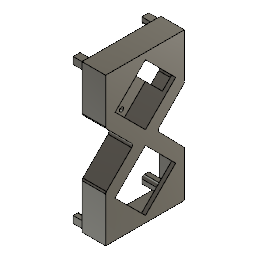
Hourglass v10 (Autodesk Fusion 360 design; units mm, degrees)
Autodesk Fusion 360 part; units mm, degrees
sketch "Sketch4" plane through (0, 0, 0) normal (1, 0, 0) x (0, 1, 0)
  line L0 (-60, 0) -> (-60, 35)
  line L1 (-60, 35) -> (0, 35)
  line L2 (0, 35) -> (0, 0)
  line L3 (-60, 0) -> (-38.7868, -21.2132)
  line L4 (-29.7466, 65.753) -> (-29.7466, -62.8744) construction
  line L5 (0, 0) -> (-20.7064, -21.2132)
  line L6 (-20.7064, -21.2132) -> (-38.7868, -21.2132)
  line L7 (-29.7466, 30) -> (-6.7656, 7.019)
  line L8 (-6.7656, 7.019) -> (-29.7466, -15.9619)
  line L9 (-29.7466, -15.9619) -> (-52.7276, 7.019)
  line L10 (-52.7276, 7.019) -> (-29.7466, 30)
  line L11 (-60, -42.4264) -> (-60, -77.4264)
  line L12 (-52.7276, -49.4454) -> (-29.7466, -72.4264)
  line L13 (-29.7466, -72.4264) -> (-6.7656, -49.4454)
  line L14 (0, -77.4264) -> (0, -42.4264)
  line L15 (-60, -42.4264) -> (-38.7868, -21.2132)
  line L16 (-6.7656, -49.4454) -> (-29.7466, -26.4645)
  line L17 (-29.7466, -26.4645) -> (-52.7276, -49.4454)
  line L18 (0, -42.4264) -> (-20.7064, -21.2132)
  line L19 (-60, -77.4264) -> (0, -77.4264)
  line L20 (-29.7466, -108.1794) -> (-29.7466, 20.448) construction
  line L21 (0, 0) -> (-13.7847, 0)
  line L22 (-45.7085, 0) -> (-60, 0)
  line L23 (0, -42.4264) -> (-13.7847, -42.4264)
  line L24 (-45.7085, -42.4264) -> (-60, -42.4264)
  line L25 (-58.8, 0.4971) -> (-58.8, 33.8)
  line L26 (-58.8, 33.8) -> (-1.2, 33.8)
  line L27 (-1.2, 33.8) -> (-1.2, 0.4886)
  line L28 (-1.2, 0.4886) -> (-22.3833, -21.2132)
  line L29 (-1.2, -42.915) -> (-22.3833, -21.2132)
  line L30 (-1.2, -76.2264) -> (-1.2, -42.915)
  line L31 (-58.8, -76.2264) -> (-1.2, -76.2264)
  line L32 (-58.8, -42.9235) -> (-58.8, -76.2264)
  line L33 (-58.8, -42.9235) -> (-37.0897, -21.2132)
  line L34 (-58.8, 0.4971) -> (-37.0897, -21.2132)
  line L35 (-29.7466, -17.659) -> (-54.4246, 7.019)
  line L36 (-54.4246, 7.019) -> (-29.7466, 31.6971)
  line L37 (-29.7466, 31.6971) -> (-5.0686, 7.019)
  line L38 (-5.0686, 7.019) -> (-29.7466, -17.659)
  line L39 (-29.7466, -24.7674) -> (-54.4246, -49.4454)
  line L40 (-54.4246, -49.4454) -> (-29.7466, -74.1235)
  line L41 (-29.7466, -74.1235) -> (-5.0686, -49.4454)
  line L42 (-5.0686, -49.4454) -> (-29.7466, -24.7674)
  line L43 (-29.7466, 30) -> (-30.5951, 30.8485)
  line L44 (-6.7656, 7.019) -> (-5.9171, 6.1705)
  line L45 (-36.8177, 22.9289) -> (-37.6662, 23.7775)
  line L46 (-13.8367, -0.052) -> (-12.9882, -0.9006)
  circle A0 centre (-31.9386, -9.5273) radius 1.6
  circle A1 centre (-46.2929, 4.827) radius 1.6
  line L47 (-6.7656, -49.4454) -> (-5.9171, -48.5969)
  line L48 (-29.7466, -72.4264) -> (-30.5951, -73.2749)
  line L49 (-13.8367, -42.3744) -> (-12.9882, -41.5258)
  line L50 (-36.8177, -65.3553) -> (-37.6662, -66.2039)
  circle A2 centre (-31.9386, -32.8991) radius 1.6
  circle A3 centre (-46.2929, -47.2534) radius 1.6
  point P0 (0, -42.4264)
  dimension "d13" = 60
  dimension "d14" = 35
  dimension "d15" = 30
  dimension "d16" = 45
  dimension "d17" = 32.5
  dimension "d18" = 45
  dimension "d19" = 5
  dimension "d20" = 32.5
  dimension "d33" = 1.2
  dimension "d34" = -1.2
  dimension "d35" = 1.2
  dimension "d50" = 10
  dimension "d51" = 10
  dimension "d58" = 3.2
  dimension "d59" = 3
  dimension "d60" = 6.1
  dimension "d61" = 3.2
  dimension "d62" = 6.1
  dimension "d63" = 3
  dimension "d66" = 10
  dimension "d67" = 10
  dimension "d72" = 3.2
  dimension "d73" = 3.2
  dimension "d74" = 6.1
  dimension "d75" = 3
  dimension "d76" = 3
  dimension "d77" = 6.1
  constraint horizontal L21
  constraint vertical L0
  constraint horizontal L1
  constraint vertical L2
  constraint coincident L2.end L5.start
  constraint perpendicular L1 L4
  constraint symmetric L3.end L4 L5.end
  constraint perpendicular L7 L8
  constraint parallel L7 L9
  constraint parallel L8 L10
  constraint coincident L4 L7.start
  constraint symmetric L2.end L6 L14.end
  constraint symmetric L2.end L6 P0
  constraint symmetric L0.start L6 L11.start
  constraint symmetric L0.end L6 L11.end
  constraint symmetric L1.end L6 L14.start
  constraint symmetric L3.end L6 L15.end
  constraint symmetric L4.start L6 L20.start
  constraint symmetric L4.end L6 L20.end
  constraint symmetric L5.end L6 L18.end
  constraint symmetric L6 L7.start L12.end
  constraint symmetric L6 L7.end L13.end
  constraint symmetric L6 L8.end L16.end
  constraint symmetric L6 L9.end L12.start
  constraint coincident L8 L21.end
  constraint collinear L21 L22
  constraint coincident L9 L22.start
  constraint coincident L16 L23.end
  constraint collinear L23 L24
  constraint coincident L17 L24.start
  constraint coincident L36 L43.end
  constraint perpendicular L36 L43
  constraint coincident L38 L44.end
  constraint perpendicular L38 L44
  constraint coincident L10 L45.start
  constraint coincident L36 L45.end
  constraint perpendicular L36 L45
  constraint coincident L8 L46.start
  constraint coincident L38 L46.end
  constraint perpendicular L38 L46
  constraint coincident L42 L47.end
  constraint perpendicular L42 L47
  constraint coincident L40 L48.end
  constraint perpendicular L40 L48
  constraint coincident L16 L49.start
  constraint coincident L42 L49.end
  constraint perpendicular L42 L49
  constraint coincident L12 L50.start
  constraint coincident L40 L50.end
  constraint perpendicular L40 L50
  measures "d13" distance of L2.end L0.start
  measures "d14" distance of L2.end L1.end
  measures "d15" distance of L0.start L3.end
  measures "d16" angle of L3 L21
  measures "d17" distance of L7.start L9.end
  measures "d18" angle of L4 L7
  measures "d19" distance of L1 L7.start
  measures "d20" distance of L7.start L7.end
  measures "d50" distance of L43 L45
  measures "d51" distance of L44 L46
  measures "d58" diameter of A0
  measures "d59" distance of L9 A0.centre
  measures "d60" distance of L8 A0.centre
  measures "d61" diameter of A1
  measures "d62" distance of L10 A1.centre
  measures "d63" distance of L9 A1.centre
  measures "d66" distance of L47 L49
  measures "d67" distance of L48 L50
  measures "d72" diameter of A2
  measures "d73" diameter of A3
  measures "d74" distance of L16 A2.centre
  measures "d75" distance of L17 A2.centre
  measures "d76" distance of L17 A3.centre
  measures "d77" distance of L12 A3.centre
extrude "Extrude2" add sketch "Sketch4" along normal blind 18 contours L3 L6 L22 L34 | L0 L1 L2 L21 L22 L25 L26 L27 L28 L34 | L6 L15 L24 L33 | L21 L22 L25 L26 L27 L28 L34 L35 L36 L37 L38 | L6 L21 L22 L28 L34 L35 L38 | L6 L23 L24 L29 L33 L39 L42 | L11 L14 L19 L23 L24 L29 L30 L31 L32 L33 | L9 L10 L22 L35 L36 L45 | L8 L9 L22 L35 L38 L46 | L5 L6 L21 L28 | L6 L18 L23 L29 | L23 L24 L29 L30 L31 L32 L33 L39 L40 L41 L42 | L16 L17 L24 L39 L42 L49 | L12 L17 L24 L39 L40 L50 | L8 L21 L38 L46 | L10 L36 L43 L45 | L8 L21 L38 L44 | L16 L23 L42 L47 | L16 L23 L42 L49 | L7 L36 L37 L38 L43 L44 | L13 L40 L41 L42 L47 L48 | L12 L40 L48 L50 makes body 1
extrude "Extrude3" add sketch "Sketch4" along normal blind 2 contours L12 L13 L16 L17 | A2 | A3 bodies 1
extrude "Extrude4" add sketch "Sketch4" along normal blind 2 contours L7 L8 L9 L10 | A0 | A1 bodies 1
fillet "Fillet1" radius 2 6 edges at (9, -38.7868, -21.2132) (9, -60, -42.4264) (9, -60, 0) (9, -20.7064, -21.2132) (9, 0, 0) (9, 0, -42.4264) on bodies 1
sketch "Sketch5" plane through (2, 0, 0) normal (1, 0, 0) x (0, 1, 0)
  line L0 (-52.7276, 7.019) -> (-29.7466, -15.9619)
  line L1 (-29.7466, -15.9619) -> (-6.7656, 7.019)
  line L2 (-6.7656, 7.019) -> (-29.7466, 30)
  line L3 (-29.7466, 30) -> (-52.7276, 7.019)
  line L4 (-36.8177, 22.9289) -> (-13.8367, -0.052)
  dimension "d29" = 10
  constraint coincident L3 L4.start
  constraint coincident L1 L4.end
  constraint perpendicular L1 L4
  measures "d29" distance of L2 L4
sketch "Sketch7" plane through (2, 0, 0) normal (1, 0, 0) x (0, 1, 0)
  line L0 (-29.7466, -26.4645) -> (-52.7276, -49.4454)
  line L1 (-52.7276, -49.4454) -> (-29.7466, -72.4264)
  line L2 (-29.7466, -72.4264) -> (-6.7656, -49.4454)
  line L3 (-6.7656, -49.4454) -> (-29.7466, -26.4645)
  line L4 (-13.8367, -42.3744) -> (-36.8177, -65.3553)
  dimension "d30" = 10
  constraint coincident L3 L4.start
  constraint perpendicular L1 L4
  constraint coincident L1 L4.end
  measures "d30" distance of L2 L4
extrude "Extrude5" cut sketch "Sketch7" sketch "Sketch5" against normal blind 2 contours L1 L2 L3 L4 of sketch 2 contours L1 L2 L3 L4 bodies 1
extrude "Extrude6" cut sketch "Sketch4" along normal blind 15 contours L21 L22 L25 L26 L27 L28 L34 L35 L36 L37 L38 | L6 L21 L22 L28 L34 L35 L38 | L6 L23 L24 L29 L33 L39 L42 | L23 L24 L29 L30 L31 L32 L33 L39 L40 L41 L42 bodies 1
extrude "Extrude8" cut sketch "Sketch4" along normal blind 15 contours L7 L36 L37 L38 L43 L44 bodies 1
fillet "Fillet4" radius 2 4 edges at (7.5, -30.5951, 30.8485) (7.5, -5.9171, 6.1705) (7.5, -54.4246, 7.019) (7.5, -29.7466, -17.659) on bodies 1
fillet "Fillet5" radius 2 2 edges at (7.5, -22.3833, -21.2132) (7.5, -37.0897, -21.2132) on bodies 1
extrude "Extrude9" cut sketch "Sketch4" along normal blind 15 contours L10 L36 L43 L45 bodies 1
extrude "Extrude10" cut sketch "Sketch4" along normal blind 15 contours L8 L21 L38 L44 bodies 1
extrude "Extrude11" cut sketch "Sketch4" along normal blind 15 contours L8 L21 L38 L46 | L8 L21 L38 L44 bodies 1
extrude "Extrude12" cut sketch "Sketch4" along normal blind 2 contours A0 | A1 bodies 1
extrude "Extrude13" cut sketch "Sketch4" along normal blind 15 contours L16 L23 L42 L47 | L16 L23 L42 L49 | L13 L40 L41 L42 L47 L48 | L12 L40 L48 L50 bodies 1
fillet "Fillet6" radius 2 2 edges at (7.5, -29.7466, -24.7674) (7.5, -54.4246, -49.4454) on bodies 1
extrude "Extrude14" cut sketch "Sketch4" along normal blind 2 contours A2 | A3 bodies 1
sketch "Sketch8" plane through (15, 0, 0) normal (-1, 0, 0) x (0, -1, 0)
  line L0 (58.8, 0.4971) -> (58.8, 33.8)
  line L1 (58.8, 33.8) -> (1.2, 33.8)
  line L2 (1.2, 33.8) -> (1.2, 0.4886)
  line L3 (1.2, 0.4886) -> (21.0197, -19.8162)
  arc A0 (21.0197, -22.6102) -> (21.0197, -19.8162) centre (19.5885, -21.2132) ccw
  line L4 (21.0197, -22.6102) -> (1.2, -42.915)
  line L5 (1.2, -42.915) -> (1.2, -76.2264)
  line L6 (1.2, -76.2264) -> (58.8, -76.2264)
  line L7 (58.8, -76.2264) -> (58.8, -42.9235)
  line L8 (58.8, -42.9235) -> (38.504, -22.6274)
  arc A1 (38.504, -19.799) -> (38.504, -22.6274) centre (39.9182, -21.2132) ccw
  line L9 (38.504, -19.799) -> (58.8, 0.4971)
  line L10 (53.0104, -50.8597) -> (37.6662, -66.2039)
  line L11 (37.6662, -66.2039) -> (36.8177, -65.3553)
  line L12 (36.8177, -65.3553) -> (29.7466, -72.4264)
  line L13 (29.7466, -72.4264) -> (6.7656, -49.4454)
  line L14 (6.7656, -49.4454) -> (13.8367, -42.3744)
  line L15 (13.8367, -42.3744) -> (12.9882, -41.5258)
  line L16 (12.9882, -41.5258) -> (28.3324, -26.1816)
  arc A2 (31.1608, -26.1816) -> (28.3324, -26.1816) centre (29.7466, -27.5958) ccw
  line L17 (31.1608, -26.1816) -> (53.0104, -48.0312)
  arc A3 (53.0104, -50.8597) -> (53.0104, -48.0312) centre (51.5962, -49.4454) ccw
  line L18 (13.8367, -0.052) -> (6.7656, 7.019)
  line L19 (6.7656, 7.019) -> (29.7466, 30)
  line L20 (29.7466, 30) -> (36.8177, 22.9289)
  line L21 (36.8177, 22.9289) -> (37.6662, 23.7775)
  line L22 (37.6662, 23.7775) -> (53.0104, 8.4332)
  arc A4 (53.0104, 5.6048) -> (53.0104, 8.4332) centre (51.5962, 7.019) ccw
  line L23 (53.0104, 5.6048) -> (31.1608, -16.2448)
  arc A5 (28.3324, -16.2448) -> (31.1608, -16.2448) centre (29.7466, -14.8306) ccw
  line L24 (28.3324, -16.2448) -> (12.9882, -0.9006)
  line L25 (12.9882, -0.9006) -> (13.8367, -0.052)
  line L26 (1.2, 33.8) -> (6.6, 33.8)
  line L27 (6.6, 33.8) -> (6.6, 28.4)
  line L28 (6.6, 28.4) -> (1.2, 28.4)
  line L29 (1.2, 28.4) -> (1.2, 33.8)
  line L30 (58.8, 33.8) -> (53.4, 33.8)
  line L31 (53.4, 33.8) -> (53.4, 28.4)
  line L32 (53.4, 28.4) -> (58.8, 28.4)
  line L33 (58.8, 28.4) -> (58.8, 33.8)
  line L34 (58.8, -76.2264) -> (53.4, -76.2264)
  line L35 (53.4, -76.2264) -> (53.4, -70.8264)
  line L36 (53.4, -70.8264) -> (58.8, -70.8264)
  line L37 (58.8, -70.8264) -> (58.8, -76.2264)
  line L38 (1.2, -76.2264) -> (6.6, -76.2264)
  line L39 (6.6, -76.2264) -> (6.6, -70.8264)
  line L40 (6.6, -70.8264) -> (1.2, -70.8264)
  line L41 (1.2, -70.8264) -> (1.2, -76.2264)
  dimension "d80" = 5.4
  dimension "d81" = 5.4
  dimension "d82" = 5.4
  dimension "d83" = 5.4
  dimension "d84" = 5.4
  dimension "d85" = 5.4
  dimension "d86" = 5.4
  dimension "d87" = 5.4
  constraint horizontal L26
  constraint vertical L27
  constraint horizontal L28
  constraint vertical L29
  constraint coincident L1.end L2.start
  constraint horizontal L30
  constraint vertical L31
  constraint horizontal L32
  constraint vertical L33
  constraint coincident L0.end L1.start
  constraint horizontal L34
  constraint vertical L35
  constraint horizontal L36
  constraint vertical L37
  constraint coincident L6.end L7.start
  constraint horizontal L38
  constraint vertical L39
  constraint horizontal L40
  constraint vertical L41
  constraint coincident L5.end L6.start
  measures "d80" distance of L1.end L26.end
  measures "d81" distance of L1.end L28.end
  measures "d82" distance of L0.end L30.end
  measures "d83" distance of L0.end L32.end
  measures "d84" distance of L6.end L34.end
  measures "d85" distance of L6.end L36.end
  measures "d86" distance of L5.end L38.end
  measures "d87" distance of L5.end L40.end
extrude "Extrude15" add sketch "Sketch8" along normal blind 15 contours L0 L1 L30 L31 L32 L33 | L1 L2 L26 L27 L28 L29 | L6 L7 L34 L35 L36 L37 | L5 L6 L38 L39 L40 L41 bodies 1
sketch "Sketch9" plane through (0, 0, 0) normal (-1, 0, 0) x (0, -1, 0)
  arc A0 (38.504, -19.799) -> (38.504, -22.6274) centre (39.9182, -21.2132) ccw
  line L0 (38.504, -22.6274) -> (58.8, -42.9235)
  line L1 (58.8, -42.9235) -> (58.8, -70.8264)
  line L2 (58.8, -70.8264) -> (53.4, -70.8264)
  line L3 (53.4, -70.8264) -> (53.4, -76.2264)
  line L4 (53.4, -76.2264) -> (6.6, -76.2264)
  line L5 (6.6, -76.2264) -> (6.6, -70.8264)
  line L6 (6.6, -70.8264) -> (1.2, -70.8264)
  line L7 (1.2, -70.8264) -> (1.2, -42.915)
  line L8 (1.2, -42.915) -> (21.0197, -22.6102)
  arc A1 (21.0197, -22.6102) -> (21.0197, -19.8162) centre (19.5885, -21.2132) ccw
  line L9 (21.0197, -19.8162) -> (1.2, 0.4886)
  line L10 (1.2, 0.4886) -> (1.2, 28.4)
  line L11 (1.2, 28.4) -> (6.6, 28.4)
  line L12 (6.6, 28.4) -> (6.6, 33.8)
  line L13 (6.6, 33.8) -> (53.4, 33.8)
  line L14 (53.4, 33.8) -> (53.4, 28.4)
  line L15 (53.4, 28.4) -> (58.8, 28.4)
  line L16 (58.8, 28.4) -> (58.8, 0.4971)
  line L17 (58.8, 0.4971) -> (38.504, -19.799)
  arc A2 (0.5688, -41.8437) -> (0, -43.2407) centre (2, -43.2407) ccw
  line L18 (0, -43.2407) -> (0, -77.4264)
  line L19 (0, -77.4264) -> (60, -77.4264)
  line L20 (60, -77.4264) -> (60, -43.2548)
  arc A3 (60, -43.2548) -> (59.4142, -41.8406) centre (58, -43.2548) ccw
  line L21 (59.4142, -41.8406) -> (40.201, -22.6274)
  arc A4 (40.201, -19.799) -> (40.201, -22.6274) centre (41.6152, -21.2132) ccw
  line L22 (40.201, -19.799) -> (59.4142, -0.5858)
  arc A5 (59.4142, -0.5858) -> (60, 0.8284) centre (58, 0.8284) ccw
  line L23 (60, 0.8284) -> (60, 35)
  line L24 (60, 35) -> (0, 35)
  line L25 (0, 35) -> (0, 0.8143)
  arc A6 (0, 0.8143) -> (0.5688, -0.5827) centre (2, 0.8143) ccw
  line L26 (0.5688, -0.5827) -> (19.3428, -19.8162)
  arc A7 (19.3428, -22.6102) -> (19.3428, -19.8162) centre (17.9116, -21.2132) ccw
  line L27 (19.3428, -22.6102) -> (0.5688, -41.8437)
  circle A8 centre (3.9, 31.1) radius 1.5
  circle A9 centre (56.1, 31.1) radius 1.5
  circle A10 centre (56.1, -73.5264) radius 1.5
  circle A11 centre (3.9, -73.5264) radius 1.5
  line L28 (6.6, 28.4) -> (1.2, 28.4)
  line L29 (1.2, 28.4) -> (1.2, 33.8)
  line L30 (1.2, 33.8) -> (6.6, 33.8)
  line L31 (6.6, 33.8) -> (6.6, 28.4)
  line L32 (53.4, 28.4) -> (58.8, 28.4)
  line L33 (58.8, 28.4) -> (58.8, 33.8)
  line L34 (58.8, 33.8) -> (53.4, 33.8)
  line L35 (53.4, 33.8) -> (53.4, 28.4)
  line L36 (53.4, -70.8264) -> (58.8, -70.8264)
  line L37 (58.8, -70.8264) -> (58.8, -76.2264)
  line L38 (58.8, -76.2264) -> (53.4, -76.2264)
  line L39 (53.4, -76.2264) -> (53.4, -70.8264)
  line L40 (6.6, -70.8264) -> (1.2, -70.8264)
  line L41 (1.2, -70.8264) -> (1.2, -76.2264)
  line L42 (1.2, -76.2264) -> (6.6, -76.2264)
  line L43 (6.6, -76.2264) -> (6.6, -70.8264)
  dimension "d90" = 3
  dimension "d91" = 2.7
  dimension "d92" = 2.7
  dimension "d93" = 3
  dimension "d94" = 2.7
  dimension "d95" = 2.7
  dimension "d96" = 3
  dimension "d97" = 2.7
  dimension "d98" = 2.7
  dimension "d99" = 3
  dimension "d100" = 2.7
  dimension "d101" = 2.7
  dimension "d195" = 5.4
  dimension "d196" = 5.4
  dimension "d197" = 5.4
  dimension "d198" = 5.4
  dimension "d199" = 5.4
  dimension "d200" = 5.4
  dimension "d201" = 5.4
  dimension "d202" = 5.4
  constraint horizontal L28
  constraint vertical L29
  constraint horizontal L30
  constraint vertical L31
  constraint coincident L11.end L12.start
  constraint horizontal L32
  constraint vertical L33
  constraint horizontal L34
  constraint vertical L35
  constraint coincident L14.end L15.start
  constraint horizontal L36
  constraint vertical L37
  constraint horizontal L38
  constraint vertical L39
  constraint coincident L2.end L3.start
  constraint horizontal L40
  constraint vertical L41
  constraint horizontal L42
  constraint vertical L43
  constraint coincident L5.end L6.start
  measures "d90" diameter of A8
  measures "d91" distance of L12 A8.centre
  measures "d92" distance of L11 A8.centre
  measures "d93" diameter of A9
  measures "d94" distance of L14 A9.centre
  measures "d95" distance of L15 A9.centre
  measures "d96" diameter of A10
  measures "d97" distance of L3 A10.centre
  measures "d98" distance of L2 A10.centre
  measures "d99" diameter of A11
  measures "d100" distance of L6 A11.centre
  measures "d101" distance of L5 A11.centre
  measures "d195" distance of L11.end L10.end
  measures "d196" distance of L11.end L12.end
  measures "d197" distance of L14.end L15.end
  measures "d198" distance of L14.end L13.end
  measures "d199" distance of L2.end L1.end
  measures "d200" distance of L2.end L3.end
  measures "d201" distance of L5.end L6.end
  measures "d202" distance of L5.end L4.end
extrude "Extrude16" cut sketch "Sketch9" against normal blind 15 contours A8 | A9 | A10 | A11 bodies 1
fillet "Fillet7" radius 2 4 edges at (7.5, -53.4, 28.4) (7.5, -53.4, -70.8264) (7.5, -6.6, 28.4) (7.5, -6.6, -70.8264) on bodies 1
fillet "Fillet8" radius 2 4 edges at (7.5, -1.2, 0.4886) (7.5, -1.2, -42.915) (7.5, -58.8, 0.4971) (7.5, -58.8, -42.9235) on bodies 1
extrude "Extrude1" add 1 faces at (0, -1.2018, 31.5424) along direction (-1, 0, 0) blind 20 separate body on bodies 1 makes body 2 in component "Lid"
sketch "Sketch10" plane through (-20, 0, 0) normal (-1, 0, 0) x (0, -1, 0)
  circle A0 centre (56.1, -73.5264) radius 1.5
  circle A1 centre (3.9, 31.1) radius 1.5
  circle A2 centre (3.9, -73.5264) radius 1.5
  circle A3 centre (56.1, 31.1) radius 1.5
  arc A4 (6.6, -72.8264) -> (4.6, -70.8264) centre (4.6, -72.8264) ccw
  line L0 (4.6, -70.8264) -> (1.2, -70.8264)
  line L1 (1.2, -70.8264) -> (1.2, -43.7293)
  arc A5 (1.7688, -42.3323) -> (1.2, -43.7293) centre (3.2, -43.7293) ccw
  line L2 (1.7688, -42.3323) -> (21.0197, -22.6102)
  arc A6 (21.0197, -22.6102) -> (21.0197, -19.8162) centre (19.5885, -21.2132) ccw
  line L3 (21.0197, -19.8162) -> (1.7688, -0.0941)
  arc A7 (1.2, 1.3029) -> (1.7688, -0.0941) centre (3.2, 1.3029) ccw
  line L4 (1.2, 1.3029) -> (1.2, 28.4)
  line L5 (1.2, 28.4) -> (4.6, 28.4)
  arc A8 (4.6, 28.4) -> (6.6, 30.4) centre (4.6, 30.4) ccw
  line L6 (6.6, 30.4) -> (6.6, 33.8)
  line L7 (6.6, 33.8) -> (53.4, 33.8)
  line L8 (53.4, 33.8) -> (53.4, 30.4)
  arc A9 (53.4, 30.4) -> (55.4, 28.4) centre (55.4, 30.4) ccw
  line L9 (55.4, 28.4) -> (58.8, 28.4)
  line L10 (58.8, 28.4) -> (58.8, 1.3255)
  arc A10 (58.2142, -0.0887) -> (58.8, 1.3255) centre (56.8, 1.3255) ccw
  line L11 (58.2142, -0.0887) -> (38.504, -19.799)
  arc A11 (38.504, -19.799) -> (38.504, -22.6274) centre (39.9182, -21.2132) ccw
  line L12 (38.504, -22.6274) -> (58.2142, -42.3377)
  arc A12 (58.8, -43.7519) -> (58.2142, -42.3377) centre (56.8, -43.7519) ccw
  line L13 (58.8, -43.7519) -> (58.8, -70.8264)
  line L14 (58.8, -70.8264) -> (55.4, -70.8264)
  arc A13 (55.4, -70.8264) -> (53.4, -72.8264) centre (55.4, -72.8264) ccw
  line L15 (53.4, -72.8264) -> (53.4, -76.2264)
  line L16 (53.4, -76.2264) -> (6.6, -76.2264)
  line L17 (6.6, -76.2264) -> (6.6, -72.8264)
  arc A14 (0.5688, -41.8437) -> (0, -43.2407) centre (2, -43.2407) ccw
  line L18 (0, -43.2407) -> (0, -77.4264)
  line L19 (0, -77.4264) -> (60, -77.4264)
  line L20 (60, -77.4264) -> (60, -43.2548)
  arc A15 (60, -43.2548) -> (59.4142, -41.8406) centre (58, -43.2548) ccw
  line L21 (59.4142, -41.8406) -> (40.201, -22.6274)
  arc A16 (40.201, -19.799) -> (40.201, -22.6274) centre (41.6152, -21.2132) ccw
  line L22 (40.201, -19.799) -> (59.4142, -0.5858)
  arc A17 (59.4142, -0.5858) -> (60, 0.8284) centre (58, 0.8284) ccw
  line L23 (60, 0.8284) -> (60, 35)
  line L24 (60, 35) -> (0, 35)
  line L25 (0, 35) -> (0, 0.8143)
  arc A18 (0, 0.8143) -> (0.5688, -0.5827) centre (2, 0.8143) ccw
  line L26 (0.5688, -0.5827) -> (19.3428, -19.8162)
  arc A19 (19.3428, -22.6102) -> (19.3428, -19.8162) centre (17.9116, -21.2132) ccw
  line L27 (19.3428, -22.6102) -> (0.5688, -41.8437)
  line L28 (0, 35) -> (60, 35)
  constraint coincident L24.end L25.start
  constraint coincident L23.end L24.start
extrude "Extrude2'" add sketch "Sketch10" along normal blind 2 contours A4 L0 L1 A5 L2 A6 L3 A7 L4 L5 A8 L6 L7 L8 A9 L9 L10 A10 L11 A11 L12 A12 L13 L14 A13 L15 L16 L17 | A14 L18 L19 L20 A15 L21 A16 L22 A17 L23 L24 L25 A18 L26 A19 L27 L28 bodies 2 in component "Lid"
sketch "Sketch11" plane through (0, 0, 0) normal (1, 0, 0) x (0, 1, 0)
  circle A0 centre (-56.1, -73.5264) radius 1.5
  circle A1 centre (-3.9, 31.1) radius 1.5
  circle A2 centre (-3.9, -73.5264) radius 1.5
  circle A3 centre (-56.1, 31.1) radius 1.5
  arc A4 (-4.6, -70.8264) -> (-6.6, -72.8264) centre (-4.6, -72.8264) ccw
  line L0 (-6.6, -72.8264) -> (-6.6, -76.2264)
  line L1 (-6.6, -76.2264) -> (-53.4, -76.2264)
  line L2 (-53.4, -76.2264) -> (-53.4, -72.8264)
  arc A5 (-53.4, -72.8264) -> (-55.4, -70.8264) centre (-55.4, -72.8264) ccw
  line L3 (-55.4, -70.8264) -> (-58.8, -70.8264)
  line L4 (-58.8, -70.8264) -> (-58.8, -43.7519)
  arc A6 (-58.2142, -42.3377) -> (-58.8, -43.7519) centre (-56.8, -43.7519) ccw
  line L5 (-58.2142, -42.3377) -> (-38.504, -22.6274)
  arc A7 (-38.504, -22.6274) -> (-38.504, -19.799) centre (-39.9182, -21.2132) ccw
  line L6 (-38.504, -19.799) -> (-58.2142, -0.0887)
  arc A8 (-58.8, 1.3255) -> (-58.2142, -0.0887) centre (-56.8, 1.3255) ccw
  line L7 (-58.8, 1.3255) -> (-58.8, 28.4)
  line L8 (-58.8, 28.4) -> (-55.4, 28.4)
  arc A9 (-55.4, 28.4) -> (-53.4, 30.4) centre (-55.4, 30.4) ccw
  line L9 (-53.4, 30.4) -> (-53.4, 33.8)
  line L10 (-53.4, 33.8) -> (-6.6, 33.8)
  line L11 (-6.6, 33.8) -> (-6.6, 30.4)
  arc A10 (-6.6, 30.4) -> (-4.6, 28.4) centre (-4.6, 30.4) ccw
  line L12 (-4.6, 28.4) -> (-1.2, 28.4)
  line L13 (-1.2, 28.4) -> (-1.2, 1.3029)
  arc A11 (-1.7688, -0.0941) -> (-1.2, 1.3029) centre (-3.2, 1.3029) ccw
  line L14 (-1.7688, -0.0941) -> (-21.0197, -19.8162)
  arc A12 (-21.0197, -19.8162) -> (-21.0197, -22.6102) centre (-19.5885, -21.2132) ccw
  line L15 (-21.0197, -22.6102) -> (-1.7688, -42.3323)
  arc A13 (-1.2, -43.7293) -> (-1.7688, -42.3323) centre (-3.2, -43.7293) ccw
  line L16 (-1.2, -43.7293) -> (-1.2, -70.8264)
  line L17 (-1.2, -70.8264) -> (-4.6, -70.8264)
  arc A14 (0, -43.2407) -> (-0.5688, -41.8437) centre (-2, -43.2407) ccw
  line L18 (-0.5688, -41.8437) -> (-19.3428, -22.6102)
  arc A15 (-19.3428, -19.8162) -> (-19.3428, -22.6102) centre (-17.9116, -21.2132) ccw
  line L19 (-19.3428, -19.8162) -> (-0.5688, -0.5827)
  arc A16 (-0.5688, -0.5827) -> (0, 0.8143) centre (-2, 0.8143) ccw
  line L20 (0, 0.8143) -> (0, 35)
  line L21 (0, 35) -> (-60, 35)
  line L22 (-60, 35) -> (-60, 0.8284)
  arc A17 (-60, 0.8284) -> (-59.4142, -0.5858) centre (-58, 0.8284) ccw
  line L23 (-59.4142, -0.5858) -> (-40.201, -19.799)
  arc A18 (-40.201, -22.6274) -> (-40.201, -19.799) centre (-41.6152, -21.2132) ccw
  line L24 (-40.201, -22.6274) -> (-59.4142, -41.8406)
  arc A19 (-59.4142, -41.8406) -> (-60, -43.2548) centre (-58, -43.2548) ccw
  line L25 (-60, -43.2548) -> (-60, -77.4264)
  line L26 (-60, -77.4264) -> (0, -77.4264)
  line L27 (0, -77.4264) -> (0, -43.2407)
  line L28 (-53.4, 33.8) -> (-58.8, 33.8)
  line L29 (-58.8, 33.8) -> (-58.8, 28.4)
  line L30 (-58.8, 28.4) -> (-53.4, 28.4)
  line L31 (-53.4, 28.4) -> (-53.4, 33.8)
  line L32 (-6.6, 33.8) -> (-1.2, 33.8)
  line L33 (-1.2, 33.8) -> (-1.2, 28.4)
  line L34 (-1.2, 28.4) -> (-6.6, 28.4)
  line L35 (-6.6, 28.4) -> (-6.6, 33.8)
  line L36 (-6.6, -76.2264) -> (-1.2, -76.2264)
  line L37 (-1.2, -76.2264) -> (-1.2, -70.8264)
  line L38 (-1.2, -70.8264) -> (-6.6, -70.8264)
  line L39 (-6.6, -70.8264) -> (-6.6, -76.2264)
  line L40 (-53.4, -76.2264) -> (-58.8, -76.2264)
  line L41 (-58.8, -76.2264) -> (-58.8, -70.8264)
  line L42 (-58.8, -70.8264) -> (-53.4, -70.8264)
  line L43 (-53.4, -70.8264) -> (-53.4, -76.2264)
  constraint horizontal L28
  constraint vertical L29
  constraint horizontal L30
  constraint vertical L31
  constraint coincident L7.end L8.start
  constraint coincident L9.end L10.start
  constraint horizontal L32
  constraint vertical L33
  constraint horizontal L34
  constraint vertical L35
  constraint coincident L12.end L13.start
  constraint coincident L10.end L11.start
  constraint horizontal L36
  constraint vertical L37
  constraint horizontal L38
  constraint vertical L39
  constraint coincident L16.end L17.start
  constraint coincident L0.end L1.start
  constraint horizontal L40
  constraint vertical L41
  constraint horizontal L42
  constraint vertical L43
  constraint coincident L3.end L4.start
  constraint coincident L1.end L2.start
chamfer "Chamfer1" distance 1 angle 45 2 edges at (-22, -2.5015, 31.6424) (-22, -54.7015, 31.6424) on bodies 2 in component "Lid"
chamfer "Chamfer2" distance 1 angle 45 2 edges at (-22, -54.7015, -72.984) (-22, -2.5015, -72.984) on bodies 2 in component "Lid"
sketch "Sketch12" plane through (-20, 0, 0) normal (1, 0, 0) x (0, 1, 0)
  line L0 (-6.6, -76.2264) -> (-6.6, -72.8264)
  arc A0 (-4.6, -70.8264) -> (-6.6, -72.8264) centre (-4.6, -72.8264) ccw
  line L1 (-4.6, -70.8264) -> (-1.2, -70.8264)
  line L2 (-1.2, -70.8264) -> (-1.2, -43.7293)
  arc A1 (-1.2, -43.7293) -> (-1.7688, -42.3323) centre (-3.2, -43.7293) ccw
  line L3 (-1.7688, -42.3323) -> (-21.0197, -22.6102)
  arc A2 (-21.0197, -19.8162) -> (-21.0197, -22.6102) centre (-19.5885, -21.2132) ccw
  line L4 (-21.0197, -19.8162) -> (-1.7688, -0.0941)
  arc A3 (-1.7688, -0.0941) -> (-1.2, 1.3029) centre (-3.2, 1.3029) ccw
  line L5 (-1.2, 1.3029) -> (-1.2, 28.4)
  line L6 (-1.2, 28.4) -> (-4.6, 28.4)
  arc A4 (-6.6, 30.4) -> (-4.6, 28.4) centre (-4.6, 30.4) ccw
  line L7 (-6.6, 30.4) -> (-6.6, 33.8)
  line L8 (-6.6, 33.8) -> (-53.4, 33.8)
  line L9 (-53.4, 33.8) -> (-53.4, 30.4)
  arc A5 (-55.4, 28.4) -> (-53.4, 30.4) centre (-55.4, 30.4) ccw
  line L10 (-55.4, 28.4) -> (-58.8, 28.4)
  line L11 (-58.8, 28.4) -> (-58.8, 1.3255)
  arc A6 (-58.8, 1.3255) -> (-58.2142, -0.0887) centre (-56.8, 1.3255) ccw
  line L12 (-58.2142, -0.0887) -> (-38.504, -19.799)
  arc A7 (-38.504, -22.6274) -> (-38.504, -19.799) centre (-39.9182, -21.2132) ccw
  line L13 (-38.504, -22.6274) -> (-58.2142, -42.3377)
  arc A8 (-58.2142, -42.3377) -> (-58.8, -43.7519) centre (-56.8, -43.7519) ccw
  line L14 (-58.8, -43.7519) -> (-58.8, -70.8264)
  line L15 (-58.8, -70.8264) -> (-55.4, -70.8264)
  arc A9 (-53.4, -72.8264) -> (-55.4, -70.8264) centre (-55.4, -72.8264) ccw
  line L16 (-53.4, -72.8264) -> (-53.4, -76.2264)
  line L17 (-53.4, -76.2264) -> (-6.6, -76.2264)
  line L18 (-52.8, 26) -> (-30.6, 26)
  line L19 (-30.6, 26) -> (-30.6, 8.5)
  line L20 (-30.6, 8.5) -> (-52.8, 8.5)
  line L21 (-52.8, 8.5) -> (-52.8, 26)
  line L22 (-31.4, 9.3) -> (-52, 9.3)
  line L23 (-52, 9.3) -> (-52, 25.2)
  line L24 (-52, 25.2) -> (-31.4, 25.2)
  line L25 (-31.4, 25.2) -> (-31.4, 9.3)
  circle A10 centre (-49.5, 22.7) radius 1.25
  circle A11 centre (-33.9, 22.7) radius 1.25
  line L26 (-46.8, -32.6464) -> (-28.62, -32.6464)
  line L27 (-28.62, -32.6464) -> (-28.62, -76.2264)
  line L28 (-28.62, -76.2264) -> (-46.8, -76.2264)
  line L29 (-46.8, -76.2264) -> (-46.8, -32.6464)
  circle A12 centre (-45.33, -34.1164) radius 0.75
  circle A13 centre (-30.09, -34.1164) radius 0.75
  circle A14 centre (-45.33, -74.7564) radius 0.75
  circle A15 centre (-30.09, -74.7564) radius 0.75
  circle A16 centre (-45.33, -34.1164) radius 1.35
  circle A17 centre (-30.09, -34.1164) radius 1.35
  circle A18 centre (-45.33, -74.7564) radius 1.35
  circle A19 centre (-30.09, -74.7564) radius 1.35
  line L30 (-26.2, -76.2264) -> (-8.2, -76.2264)
  line L31 (-8.2, -76.2264) -> (-8.2, -47.7264)
  line L32 (-8.2, -47.7264) -> (-26.2, -47.7264)
  line L33 (-26.2, -47.7264) -> (-26.2, -76.2264)
  line L34 (-27, -77.0264) -> (-7.4, -77.0264)
  line L35 (-7.4, -77.0264) -> (-7.4, -46.9264)
  line L36 (-7.4, -46.9264) -> (-27, -46.9264)
  line L37 (-27, -46.9264) -> (-27, -77.0264)
  line L38 (-23.2, -46.9264) -> (-23.2, -47.7264)
  line L39 (-11.2, -47.7264) -> (-11.2, -46.9264)
  line L40 (-20.6, 27.8) -> (-11.6, 27.8)
  line L41 (-11.6, 27.8) -> (-11.6, 31.8)
  line L42 (-11.6, 31.8) -> (-20.6, 31.8)
  line L43 (-20.6, 31.8) -> (-20.6, 27.8)
  dimension "d115" = 22.2
  dimension "d116" = 17.5
  dimension "d117" = 6
  dimension "d118" = 0.8
  dimension "d119" = 2.5
  dimension "d120" = 2.5
  dimension "d121" = 2.5
  dimension "d122" = 2.5
  dimension "d123" = 2.5
  dimension "d124" = 2.5
  dimension "d131" = 18.18
  dimension "d132" = 43.58
  dimension "d133" = 12
  dimension "d134" = 1.5
  dimension "d135" = 1.47
  dimension "d136" = 1.47
  dimension "d137" = 1.5
  dimension "d138" = 1.5
  dimension "d139" = 1.5
  dimension "d140" = 1.47
  dimension "d141" = 1.47
  dimension "d142" = 1.47
  dimension "d143" = 1.47
  dimension "d144" = 1.47
  dimension "d145" = 1.47
  dimension "d146" = 2.7
  dimension "d147" = 2.7
  dimension "d148" = 2.7
  dimension "d149" = 2.7
  dimension "d168" = 18
  dimension "d169" = 28.5
  dimension "d170" = 7
  dimension "d171" = 0.8
  dimension "d172" = 3.8
  dimension "d173" = 3.8
  dimension "d211" = 9
  dimension "d212" = 4
  dimension "d213" = 5
  dimension "d214" = 2
  constraint horizontal L18
  constraint vertical L19
  constraint horizontal L20
  constraint vertical L21
  constraint horizontal L26
  constraint vertical L27
  constraint horizontal L28
  constraint vertical L29
  constraint collinear L17 L28
  constraint concentric A12 A16
  constraint concentric A13 A17
  constraint concentric A14 A18
  constraint concentric A15 A19
  constraint horizontal L30
  constraint vertical L31
  constraint horizontal L32
  constraint vertical L33
  constraint coincident L17 L30.start
  constraint coincident L36 L38.start
  constraint coincident L32 L38.end
  constraint perpendicular L32 L38
  constraint coincident L32 L39.start
  constraint coincident L36 L39.end
  constraint perpendicular L36 L39
  constraint horizontal L40
  constraint vertical L41
  constraint horizontal L42
  constraint vertical L43
  measures "d115" distance of L18.start L18.end
  measures "d116" distance of L18.start L20.end
  measures "d117" distance of L11 L21
  measures "d119" diameter of A10
  measures "d120" diameter of A11
  measures "d121" distance of L23 A10.centre
  measures "d122" distance of L24 A10.centre
  measures "d123" distance of L25 A11.centre
  measures "d124" distance of L24 A11.centre
  measures "d131" distance of L26.start L26.end
  measures "d132" distance of L26.start L28.end
  measures "d133" distance of L14 L29
  measures "d134" diameter of A12
  measures "d135" distance of L29 A12.centre
  measures "d136" distance of L26 A12.centre
  measures "d137" diameter of A13
  measures "d138" diameter of A14
  measures "d139" diameter of A15
  measures "d140" distance of L29 A14.centre
  measures "d141" distance of L28 A14.centre
  measures "d142" distance of L27 A15.centre
  measures "d143" distance of L28 A15.centre
  measures "d144" distance of L27 A13.centre
  measures "d145" distance of L26 A13.centre
  measures "d146" diameter of A16
  measures "d147" diameter of A17
  measures "d148" diameter of A18
  measures "d149" diameter of A19
  measures "d168" distance of L30.start L30.end
  measures "d169" distance of L30.start L32.end
  measures "d170" distance of L2 L31
  measures "d172" distance of L37 L38
  measures "d173" distance of L35 L39
  measures "d211" distance of L40.start L40.end
  measures "d212" distance of L40.start L42.end
  measures "d213" distance of L7 L41
  measures "d214" distance of L8 L42
extrude "Extrude3'" add sketch "Sketch12" along normal blind 6 contours L18 L19 L20 L21 bodies 2 in component "Lid"
extrude "Extrude4'" add sketch "Sketch12" along normal blind 4 contours L22 L23 L24 L25 bodies 2 in component "Lid"
extrude "Extrude5'" cut 1 faces at (-14, -45.1333, 25.7333) along direction (-1, 0, 0) blind 0.5 on bodies 2 bodies 2 in component "Lid"
extrude "Extrude6'" add sketch "Sketch12" along normal blind 5 contours A16 | A17 | A18 | A19 bodies 2 in component "Lid"
sketch "Sketch14" plane through (0, 0, -76.2264) normal (0, 0, 1) x (-1, 0, 0)
  line L0 (0, 53.4) -> (0, 6.6)
  line L1 (0, 6.6) -> (20, 6.6)
  line L2 (20, 6.6) -> (20, 53.4)
  line L3 (20, 53.4) -> (0, 53.4)
  line L4 (15, 44) -> (15, 31.5) construction
  line L5 (10.75, 40.585) -> (10.75, 34.835)
  arc A0 (10.75, 34.835) -> (13.5, 34.835) centre (12.125, 34.835) ccw
  line L6 (13.5, 34.835) -> (13.5, 40.585)
  arc A1 (13.5, 40.585) -> (10.75, 40.585) centre (12.125, 40.585) ccw
  line L7 (12.125, 41.96) -> (12.125, 33.46) construction
  line L8 (10.75, 37.71) -> (13.5, 37.71) construction
  line L9 (13.5, 14.325) -> (13.5, 20.075)
  arc A2 (13.5, 20.075) -> (10.75, 20.075) centre (12.125, 20.075) ccw
  line L10 (10.75, 20.075) -> (10.75, 14.325)
  arc A3 (10.75, 14.325) -> (13.5, 14.325) centre (12.125, 14.325) ccw
  line L11 (12.125, 12.95) -> (12.125, 21.45) construction
  line L12 (13.5, 17.2) -> (10.75, 17.2) construction
  dimension "d161" = 2.75
  dimension "d162" = 8.5
  dimension "d163" = 4.25
  dimension "d164" = 15.69
  dimension "d165" = 6.5
  dimension "d182" = 8.5
  dimension "d183" = 2.75
  dimension "d184" = 4.25
  dimension "d185" = 10.6
  dimension "d186" = 6.5
  constraint vertical L4
  constraint tangent L5 A0
  constraint tangent A0 L6
  constraint parallel L5 L6
  constraint tangent L6 A1
  constraint tangent L5 A1
  constraint midpoint A1 L7.start
  constraint midpoint A0 L7.end
  constraint parallel L4 L7
  constraint coincident L5 L8.start
  constraint coincident L6 L8.end
  constraint perpendicular L6 L8
  constraint tangent L9 A2
  constraint tangent A2 L10
  constraint parallel L9 L10
  constraint tangent L10 A3
  constraint tangent L9 A3
  constraint midpoint A3 L11.start
  constraint midpoint A2 L11.end
  constraint vertical L11
  constraint coincident L9 L12.start
  constraint coincident L10 L12.end
  constraint perpendicular L10 L12
  measures "d161" diameter of A0
  measures "d162" distance of L7.start L7.end
  measures "d163" distance of L7.start L8
  measures "d164" distance of L3 L8
  measures "d165" distance of L2 L6
  measures "d182" distance of L11.start L11.end
  measures "d183" distance of L9 L10
  measures "d184" distance of L11.end L12
  measures "d185" distance of L1 L12
  measures "d186" distance of L2 L9
extrude "Extrude8'" cut sketch "Sketch14" against normal blind 2 contours L5 A0 L6 A1 bodies 2 in component "Lid"
extrude "Extrude9'" add 1 faces at (-16, -39.3598, 13.4409) along direction (1, 0, 0) blind 1 on bodies 2 bodies 2 in component "Lid"
extrude "Extrude10'" add 1 faces at (-14.5, -45.1333, 25.7333) along direction (1, 0, 0) blind 1 on bodies 2 bodies 2 in component "Lid"
extrude "Extrude11'" add sketch "Sketch12" along normal blind 6.5 contours L17 L31 L32 L35 L36 L39 | L17 L32 L33 L36 L37 L38 bodies 2 in component "Lid"
extrude "Extrude12'" add sketch "Sketch12" along normal blind 5 contours L17 L30 L31 L32 L33 | L32 L36 L38 L39 bodies 2 in component "Lid"
extrude "Extrude15'" add 1 faces at (-15, -15.2, -66.7264) along direction (1, 0, 0) blind 0.25 on bodies 2 bodies 2 in component "Lid"
extrude "Extrude16'" cut sketch "Sketch14" against normal blind 2 contours L9 A2 L10 A3 bodies 2 in component "Lid"
extrude "Extrude17" add sketch "Sketch9" along normal blind 8 contours L14 L15 L32 L33 L34 L35 | L2 L3 L36 L37 L38 L39 | L11 L12 L28 L29 L30 L31 | L5 L6 L40 L41 L42 L43 bodies 1
fillet "Fillet9" radius 2 4 edges at (-4, -6.6, -70.8264) (-4, -6.6, 28.4) (-4, -53.4, 28.4) (-4, -53.4, -70.8264) on bodies 1
extrude "Extrude17'" cut sketch "Sketch11" against normal blind 8 contours A4 L0 L17 L36 L37 L38 L39 bodies 2 in component "Lid"
extrude "Extrude18" cut sketch "Sketch11" against normal blind 8 contours L2 A5 L3 L40 L41 L42 L43 | L11 A10 L12 L32 L33 L34 L35 | L8 A9 L9 L28 L29 L30 L31 bodies 2 in component "Lid"
extrude "Extrude19" cut sketch "Sketch12" against normal blind 2 contours L40 L41 L42 L43 bodies 2 in component "Lid"
component "Lid" placed x (1, 0, 0) y (0, 1, 0) z (0, 0, 1) at (0, 0, 0)
equation "d91 = 1.2 mm + 1.5 mm"
equation "d92 = 1.2 mm + 1.5 mm"
equation "d115 = 21.4 mm + 0.8 mm"
equation "d163 = ( 8.5 / 2 ) * 1 mm"
equation "d164 = 9.42 mm + ( 12.54 / 2 ) * 1 mm"
equation "d165 = 5 mm + 1.5 mm"
equation "d185 = 1.6 mm + 9 mm"
